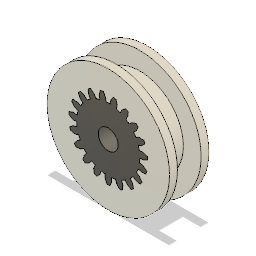
bobin v1 (Autodesk Fusion 360 design; units mm, degrees)
description: Spur Gear; Module: 12.7; Num Teeth: 19; Pressure Angle: 20.0; Backlash: 0.15 mm
Autodesk Fusion 360 part; units mm, degrees
sketch "Sketch1" plane through (0, 0, 0) normal (0, 0, 1) x (1, 0, 0) in component "Spur Gear (19 teeth)"
  circle A0 centre (0, 0) radius 105.3592
  circle A1 centre (0, 0) radius 2.5
extrude "Extrude1" add sketch "Sketch1" along normal blind 10 makes body 1 in component "Spur Gear (19 teeth)"
sketch "Sketch2" plane through (0, 0, 0) normal (0, 0, 1) x (1, 0, 0) in component "Spur Gear (19 teeth)"
  spline S0 degree 5 poles (112.838, -11.0102) (112.8973, -11.0159) (113.0158, -11.0259) (113.1938, -11.0359) (113.4315, -11.04) (113.7289, -11.0326) (114.0267, -11.0162) (114.3246, -10.9942) (114.6226, -10.9694) (114.9207, -10.9425) (115.2187, -10.9134) (115.5167, -10.8815) (115.8147, -10.8457) (116.1127, -10.8055) (116.4106, -10.7609) (116.7084, -10.7123) (117.0062, -10.6603) (117.3038, -10.6054) (117.6013, -10.548) (117.8987, -10.4882) (118.1959, -10.4261) (118.4929, -10.3614) (118.7898, -10.294) (119.0865, -10.2239) (119.3831, -10.1512) (119.6794, -10.0758) (119.9755, -9.9981) (120.2715, -9.918) (120.5672, -9.8357) (120.8627, -9.7512) (121.158, -9.6646) (121.453, -9.5758) (121.7478, -9.4848) (122.0423, -9.3917) (122.3366, -9.2964) (122.6306, -9.199) (122.9244, -9.0996) (123.2178, -8.9982) (123.5111, -8.8949) (123.804, -8.7896) (124.0966, -8.6823) (124.3889, -8.5732) (124.681, -8.4621) (124.9727, -8.3492) (125.2641, -8.2344) (125.5552, -8.1178) (125.846, -7.9993) (126.1365, -7.879) (126.4266, -7.757) (126.7164, -7.6332) (127.0059, -7.5077) (127.295, -7.3804) (127.5837, -7.2514) (127.8722, -7.1207) (128.1602, -6.9883) (128.4479, -6.8542) (128.7353, -6.7185) (129.0222, -6.5811) (129.3088, -6.4421) (129.595, -6.3015) (129.8809, -6.1592) (130.1663, -6.0154) (130.4514, -5.8699) (130.7361, -5.7229) (131.0203, -5.5743) (131.3042, -5.4242) (131.5877, -5.2725) (131.8707, -5.1193) (132.1534, -4.9646) (132.4356, -4.8083) (132.7174, -4.6506) (132.9425, -4.5232) (133.1112, -4.4269) (133.2235, -4.3625) (133.2797, -4.3302) knots 0 0 0 0 0 0 0.01428571 0.02857143 0.04285714 0.05714286 0.07142857 0.08571429 0.1 0.11428571 0.12857143 0.14285714 0.15714286 0.17142857 0.18571429 0.2 0.21428571 0.22857143 0.24285714 0.25714286 0.27142857 0.28571429 0.3 0.31428571 0.32857143 0.34285714 0.35714286 0.37142857 0.38571429 0.4 0.41428571 0.42857143 0.44285714 0.45714286 0.47142857 0.48571429 0.5 0.51428571 0.52857143 0.54285714 0.55714286 0.57142857 0.58571429 0.6 0.61428571 0.62857143 0.64285714 0.65714286 0.67142857 0.68571429 0.7 0.71428571 0.72857143 0.74285714 0.75714286 0.77142857 0.78571429 0.8 0.81428571 0.82857143 0.84285714 0.85714286 0.87142857 0.88571429 0.9 0.91428571 0.92857143 0.94285714 0.95714286 0.97142857 0.98571429 1 1 1 1 1 1
  spline S1 degree 5 poles (112.838, 11.0102) (112.8973, 11.0159) (113.0158, 11.0259) (113.1938, 11.0359) (113.4315, 11.04) (113.7289, 11.0326) (114.0267, 11.0162) (114.3246, 10.9942) (114.6226, 10.9694) (114.9207, 10.9425) (115.2187, 10.9134) (115.5167, 10.8815) (115.8147, 10.8457) (116.1127, 10.8055) (116.4106, 10.7609) (116.7084, 10.7123) (117.0062, 10.6603) (117.3038, 10.6054) (117.6013, 10.548) (117.8987, 10.4882) (118.1959, 10.4261) (118.4929, 10.3614) (118.7898, 10.294) (119.0865, 10.2239) (119.3831, 10.1512) (119.6794, 10.0758) (119.9755, 9.9981) (120.2715, 9.918) (120.5672, 9.8357) (120.8627, 9.7512) (121.158, 9.6646) (121.453, 9.5758) (121.7478, 9.4848) (122.0423, 9.3917) (122.3366, 9.2964) (122.6306, 9.199) (122.9244, 9.0996) (123.2178, 8.9982) (123.5111, 8.8949) (123.804, 8.7896) (124.0966, 8.6823) (124.3889, 8.5732) (124.681, 8.4621) (124.9727, 8.3492) (125.2641, 8.2344) (125.5552, 8.1178) (125.846, 7.9993) (126.1365, 7.879) (126.4266, 7.757) (126.7164, 7.6332) (127.0059, 7.5077) (127.295, 7.3804) (127.5837, 7.2514) (127.8722, 7.1207) (128.1602, 6.9883) (128.4479, 6.8542) (128.7353, 6.7185) (129.0222, 6.5811) (129.3088, 6.4421) (129.595, 6.3015) (129.8809, 6.1592) (130.1663, 6.0154) (130.4514, 5.8699) (130.7361, 5.7229) (131.0203, 5.5743) (131.3042, 5.4242) (131.5877, 5.2725) (131.8707, 5.1193) (132.1534, 4.9646) (132.4356, 4.8083) (132.7174, 4.6506) (132.9425, 4.5232) (133.1112, 4.4269) (133.2235, 4.3625) (133.2797, 4.3302) knots 0 0 0 0 0 0 0.01428571 0.02857143 0.04285714 0.05714286 0.07142857 0.08571429 0.1 0.11428571 0.12857143 0.14285714 0.15714286 0.17142857 0.18571429 0.2 0.21428571 0.22857143 0.24285714 0.25714286 0.27142857 0.28571429 0.3 0.31428571 0.32857143 0.34285714 0.35714286 0.37142857 0.38571429 0.4 0.41428571 0.42857143 0.44285714 0.45714286 0.47142857 0.48571429 0.5 0.51428571 0.52857143 0.54285714 0.55714286 0.57142857 0.58571429 0.6 0.61428571 0.62857143 0.64285714 0.65714286 0.67142857 0.68571429 0.7 0.71428571 0.72857143 0.74285714 0.75714286 0.77142857 0.78571429 0.8 0.81428571 0.82857143 0.84285714 0.85714286 0.87142857 0.88571429 0.9 0.91428571 0.92857143 0.94285714 0.95714286 0.97142857 0.98571429 1 1 1 1 1 1
  arc A0 (133.2797, -4.3302) -> (133.2797, 4.3302) centre (0, 0) ccw
  line L0 (104.8512, -10.2318) -> (112.838, -11.0102)
  line L1 (104.8512, 10.2318) -> (112.838, 11.0102)
  line L2 (104.8512, -10.2318) -> (104.8512, 10.2318)
  point P0 (114.2728, -10.9975)
  point P1 (115.7195, -10.8565)
  point P2 (117.1734, -10.6291)
  point P3 (118.6325, -10.3293)
  point P4 (120.0955, -9.9653)
  point P5 (121.5612, -9.5421)
  point P6 (123.0286, -9.0634)
  point P7 (124.4968, -8.5319)
  point P8 (125.9651, -7.9498)
  point P9 (127.4326, -7.3187)
  point P10 (128.8985, -6.6401)
  point P11 (130.3621, -5.9152)
  point P12 (131.8228, -5.145)
  point P13 (114.2728, 10.9975)
  point P14 (115.7195, 10.8565)
  point P15 (117.1734, 10.6291)
  point P16 (118.6325, 10.3293)
  point P17 (120.0955, 9.9653)
  point P18 (121.5612, 9.5421)
  point P19 (123.0286, 9.0634)
  point P20 (124.4968, 8.5319)
  point P21 (125.9651, 7.9498)
  point P22 (127.4326, 7.3187)
  point P23 (128.8985, 6.6401)
  point P24 (130.3621, 5.9152)
  point P25 (131.8228, 5.145)
extrude "Extrude2" add sketch "Sketch2" along normal blind 10 bodies 1 in component "Spur Gear (19 teeth)"
fillet "Fillet1" radius 0.75 2 edges at (104.8611, -10.2328, 5) (104.8611, 10.2328, 5) on bodies 1 in component "Spur Gear (19 teeth)"
pattern_circular "C-Pattern1" count 19 over 360 about axis through (0, 0, 0) along (0, 0, 1) of "Extrude2", "Fillet1" in component "Spur Gear (19 teeth)"
sketch "Sketch3" plane through (0, 0, 0) normal (0, 0, 1) x (1, 0, 0) in component "Spur Gear (19 teeth)"
  circle A0 centre (0, 0) radius 120.65 construction
sketch "Sketch2 (2)" plane through (0, 0, 0) normal (0, 0, 1) x (1, 0, 0)
  circle A0 centre (0, 66.5) radius 8
  line L0 (0.8502, 58.5453) -> (0.8502, 57.6)
  line L1 (0.8502, 57.6) -> (0.3705, 56.5344)
  line L2 (0.3705, 56.5344) -> (-0.3738, 56.5344)
  line L3 (-0.3738, 56.5344) -> (-0.8, 57.6)
  line L4 (-0.8, 57.6) -> (-0.8, 58.5401)
  line L5 (2.1332, 57.8225) -> (1.8279, 58.7116)
  line L6 (2.8823, 56.953) -> (2.1332, 57.8225)
  line L7 (3.5862, 57.1947) -> (2.8823, 56.953)
  line L8 (3.694, 58.3583) -> (3.5862, 57.1947)
  line L9 (3.3871, 59.2524) -> (3.694, 58.3583)
  line L10 (4.8352, 58.9853) -> (4.2578, 59.7272)
  line L11 (5.826, 58.4062) -> (4.8352, 58.9853)
  line L12 (6.4133, 58.8633) -> (5.826, 58.4062)
  line L13 (6.1375, 59.9989) -> (6.4133, 58.8633)
  line L14 (5.5568, 60.7449) -> (6.1375, 59.9989)
  line L15 (7.0132, 60.9624) -> (6.2262, 61.4766)
  line L16 (8.1384, 60.7364) -> (7.0132, 60.9624)
  line L17 (8.5455, 61.3595) -> (8.1384, 60.7364)
  line L18 (7.9158, 62.344) -> (8.5455, 61.3595)
  line L19 (7.1244, 62.861) -> (7.9158, 62.344)
  line L20 (8.4313, 63.5397) -> (7.5199, 63.7704)
  line L21 (9.5689, 63.6913) -> (8.4313, 63.5397)
  line L22 (9.7516, 64.4127) -> (9.5689, 63.6913)
  line L23 (8.8364, 65.1394) -> (9.7516, 64.4127)
  line L24 (7.92, 65.3715) -> (8.8364, 65.1394)
  line L25 (8.9357, 66.4377) -> (7.9988, 66.3601)
  line L26 (9.9624, 66.9505) -> (8.9357, 66.4377)
  line L27 (9.901, 67.6922) -> (9.9624, 66.9505)
  line L28 (8.7994, 68.0823) -> (9.901, 67.6922)
  line L29 (7.8573, 68.0042) -> (8.7994, 68.0823)
  line L30 (8.4717, 69.3425) -> (7.6108, 68.9648)
  line L31 (9.2764, 70.1608) -> (8.4717, 69.3425)
  line L32 (8.9774, 70.8424) -> (9.2764, 70.1608)
  line L33 (7.8088, 70.8537) -> (8.9774, 70.8424)
  line L34 (6.9432, 70.474) -> (7.8088, 70.8537)
  line L35 (7.0898, 71.9392) -> (6.3981, 71.3025)
  line L36 (7.5851, 72.9745) -> (7.0898, 71.9392)
  line L37 (7.081, 73.5221) -> (7.5851, 72.9745)
  line L38 (5.9721, 73.1534) -> (7.081, 73.5221)
  line L39 (5.2766, 72.5131) -> (5.9721, 73.1534)
  line L40 (4.9395, 73.9466) -> (4.4921, 73.1198)
  line L41 (5.0718, 75.0866) -> (4.9395, 73.9466)
  line L42 (4.4173, 75.4408) -> (5.0718, 75.0866)
  line L43 (3.4882, 74.732) -> (4.4173, 75.4408)
  line L44 (3.0382, 73.9006) -> (3.4882, 74.732)
  line L45 (2.254, 75.1469) -> (2.0992, 74.2197)
  line L46 (2.0089, 76.2682) -> (2.254, 75.1469)
  line L47 (1.2749, 76.3907) -> (2.0089, 76.2682)
  line L48 (0.6262, 75.4186) -> (1.2749, 76.3907)
  line L49 (0.4706, 74.4861) -> (0.6262, 75.4186)
  line L50 (-0.6758, 75.4103) -> (-0.5211, 74.483)
  line L51 (-1.2716, 76.3912) -> (-0.6758, 75.4103)
  line L52 (-2.0057, 76.2687) -> (-1.2716, 76.3912)
  line L53 (-2.3035, 75.1387) -> (-2.0057, 76.2687)
  line L54 (-2.148, 74.2063) -> (-2.3035, 75.1387)
  line L55 (-3.5324, 74.7081) -> (-3.0849, 73.8813)
  line L56 (-4.4144, 75.4424) -> (-3.5324, 74.7081)
  line L57 (-5.0689, 75.0882) -> (-4.4144, 75.4424)
  line L58 (-4.9837, 73.9226) -> (-5.0689, 75.0882)
  line L59 (-4.5338, 73.0913) -> (-4.9837, 73.9226)
  line L60 (-6.0061, 73.1164) -> (-5.3145, 72.4797)
  line L61 (-7.0788, 73.5245) -> (-6.0061, 73.1164)
  line L62 (-7.5828, 72.9769) -> (-7.0788, 73.5245)
  line L63 (-7.1238, 71.9023) -> (-7.5828, 72.9769)
  line L64 (-6.4283, 71.262) -> (-7.1238, 71.9023)
  line L65 (-7.829, 70.8077) -> (-6.9681, 70.4301)
  line L66 (-8.9761, 70.8454) -> (-7.829, 70.8077)
  line L67 (-9.275, 70.1639) -> (-8.9761, 70.8454)
  line L68 (-8.4919, 69.2965) -> (-9.275, 70.1639)
  line L69 (-7.6262, 68.9167) -> (-8.4919, 69.2965)
  line L70 (-8.8035, 68.0322) -> (-7.8666, 67.9546)
  line L71 (-9.9007, 67.6954) -> (-8.8035, 68.0322)
  line L72 (-9.9621, 66.9537) -> (-9.9007, 67.6954)
  line L73 (-8.9398, 66.3876) -> (-9.9621, 66.9537)
  line L74 (-7.9977, 66.3096) -> (-8.9398, 66.3876)
  line L75 (-8.8241, 65.0907) -> (-7.9127, 65.3215)
  line L76 (-9.7524, 64.4159) -> (-8.8241, 65.0907)
  line L77 (-9.5697, 63.6945) -> (-9.7524, 64.4159)
  line L78 (-8.4189, 63.4909) -> (-9.5697, 63.6945)
  line L79 (-7.5026, 63.723) -> (-8.4189, 63.4909)
  line L80 (-7.8883, 62.3019) -> (-7.1013, 62.8161)
  line L81 (-8.5473, 61.3622) -> (-7.8883, 62.3019)
  line L82 (-8.1402, 60.7392) -> (-8.5473, 61.3622)
  line L83 (-6.9857, 60.9204) -> (-8.1402, 60.7392)
  line L84 (-6.1944, 61.4374) -> (-6.9857, 60.9204)
  line L85 (-6.0978, 59.968) -> (-5.5204, 60.7099)
  line L86 (-6.4159, 58.8653) -> (-6.0978, 59.968)
  line L87 (-5.8286, 58.4082) -> (-6.4159, 58.8653)
  line L88 (-4.7955, 58.9544) -> (-5.8286, 58.4082)
  line L89 (-4.2149, 59.7004) -> (-4.7955, 58.9544)
  line L90 (-3.6465, 58.342) -> (-3.3412, 59.2312)
  line L91 (-3.5893, 57.1957) -> (-3.6465, 58.342)
  line L92 (-2.8854, 56.9541) -> (-3.5893, 57.1957)
  line L93 (-2.0856, 57.8062) -> (-2.8854, 56.9541)
  line L94 (-1.7787, 58.7002) -> (-2.0856, 57.8062)
  dimension "d15" = 16
  dimension "d19" = 360
  constraint coincident A0 L0.start
  constraint vertical L0
  constraint perpendicular L0 L2
  constraint coincident A0 L4.end
  constraint perpendicular L2 L4
  measures "d15" diameter of A0
extrude "Extrude1'" add sketch "Sketch2 (2)" along normal blind 10 separate body makes body 2
sketch "Sketch3 (2)" plane through (0, 0, 10) normal (0, 0, 1) x (1, 0, 0)
  arc A0 (0.8502, 58.5453) -> (1.8279, 58.7116) centre (0, 66.5) ccw
  line L0 (1.8279, 58.7116) -> (2.1332, 57.8225)
  line L1 (2.1332, 57.8225) -> (2.8823, 56.953)
  line L2 (2.8823, 56.953) -> (3.5862, 57.1947)
  line L3 (3.5862, 57.1947) -> (3.694, 58.3583)
  line L4 (3.694, 58.3583) -> (3.3871, 59.2524)
  arc A1 (3.3871, 59.2524) -> (4.2578, 59.7272) centre (0, 66.5) ccw
  line L5 (4.2578, 59.7272) -> (4.8352, 58.9853)
  line L6 (4.8352, 58.9853) -> (5.826, 58.4062)
  line L7 (5.826, 58.4062) -> (6.4133, 58.8633)
  line L8 (6.4133, 58.8633) -> (6.1375, 59.9989)
  line L9 (6.1375, 59.9989) -> (5.5568, 60.7449)
  arc A2 (5.5568, 60.7449) -> (6.2262, 61.4766) centre (0, 66.5) ccw
  line L10 (6.2262, 61.4766) -> (7.0132, 60.9624)
  line L11 (7.0132, 60.9624) -> (8.1384, 60.7364)
  line L12 (8.1384, 60.7364) -> (8.5455, 61.3595)
  line L13 (8.5455, 61.3595) -> (7.9158, 62.344)
  line L14 (7.9158, 62.344) -> (7.1244, 62.861)
  arc A3 (7.1244, 62.861) -> (7.5199, 63.7704) centre (0, 66.5) ccw
  line L15 (7.5199, 63.7704) -> (8.4313, 63.5397)
  line L16 (8.4313, 63.5397) -> (9.5689, 63.6913)
  line L17 (9.5689, 63.6913) -> (9.7516, 64.4127)
  line L18 (9.7516, 64.4127) -> (8.8364, 65.1394)
  line L19 (8.8364, 65.1394) -> (7.92, 65.3715)
  arc A4 (7.92, 65.3715) -> (7.9988, 66.3601) centre (0, 66.5) ccw
  line L20 (7.9988, 66.3601) -> (8.9357, 66.4377)
  line L21 (8.9357, 66.4377) -> (9.9624, 66.9505)
  line L22 (9.9624, 66.9505) -> (9.901, 67.6922)
  line L23 (9.901, 67.6922) -> (8.7994, 68.0823)
  line L24 (8.7994, 68.0823) -> (7.8573, 68.0042)
  arc A5 (7.8573, 68.0042) -> (7.6108, 68.9648) centre (0, 66.5) ccw
  line L25 (7.6108, 68.9648) -> (8.4717, 69.3425)
  line L26 (8.4717, 69.3425) -> (9.2764, 70.1608)
  line L27 (9.2764, 70.1608) -> (8.9774, 70.8424)
  line L28 (8.9774, 70.8424) -> (7.8088, 70.8537)
  line L29 (7.8088, 70.8537) -> (6.9432, 70.474)
  arc A6 (6.9432, 70.474) -> (6.3981, 71.3025) centre (0, 66.5) ccw
  line L30 (6.3981, 71.3025) -> (7.0898, 71.9392)
  line L31 (7.0898, 71.9392) -> (7.5851, 72.9745)
  line L32 (7.5851, 72.9745) -> (7.081, 73.5221)
  line L33 (7.081, 73.5221) -> (5.9721, 73.1534)
  line L34 (5.9721, 73.1534) -> (5.2766, 72.5131)
  arc A7 (5.2766, 72.5131) -> (4.4921, 73.1198) centre (0, 66.5) ccw
  line L35 (4.4921, 73.1198) -> (4.9395, 73.9466)
  line L36 (4.9395, 73.9466) -> (5.0718, 75.0866)
  line L37 (5.0718, 75.0866) -> (4.4173, 75.4408)
  line L38 (4.4173, 75.4408) -> (3.4882, 74.732)
  line L39 (3.4882, 74.732) -> (3.0382, 73.9006)
  arc A8 (3.0382, 73.9006) -> (2.0992, 74.2197) centre (0, 66.5) ccw
  line L40 (2.0992, 74.2197) -> (2.254, 75.1469)
  line L41 (2.254, 75.1469) -> (2.0089, 76.2682)
  line L42 (2.0089, 76.2682) -> (1.2749, 76.3907)
  line L43 (1.2749, 76.3907) -> (0.6262, 75.4186)
  line L44 (0.6262, 75.4186) -> (0.4706, 74.4861)
  arc A9 (0.4706, 74.4861) -> (-0.5211, 74.483) centre (0, 66.5) ccw
  line L45 (-0.5211, 74.483) -> (-0.6758, 75.4103)
  line L46 (-0.6758, 75.4103) -> (-1.2716, 76.3912)
  line L47 (-1.2716, 76.3912) -> (-2.0057, 76.2687)
  line L48 (-2.0057, 76.2687) -> (-2.3035, 75.1387)
  line L49 (-2.3035, 75.1387) -> (-2.148, 74.2063)
  arc A10 (-2.148, 74.2063) -> (-3.0849, 73.8813) centre (0, 66.5) ccw
  line L50 (-3.0849, 73.8813) -> (-3.5324, 74.7081)
  line L51 (-3.5324, 74.7081) -> (-4.4144, 75.4424)
  line L52 (-4.4144, 75.4424) -> (-5.0689, 75.0882)
  line L53 (-5.0689, 75.0882) -> (-4.9837, 73.9226)
  line L54 (-4.9837, 73.9226) -> (-4.5338, 73.0913)
  arc A11 (-4.5338, 73.0913) -> (-5.3145, 72.4797) centre (0, 66.5) ccw
  line L55 (-5.3145, 72.4797) -> (-6.0061, 73.1164)
  line L56 (-6.0061, 73.1164) -> (-7.0788, 73.5245)
  line L57 (-7.0788, 73.5245) -> (-7.5828, 72.9769)
  line L58 (-7.5828, 72.9769) -> (-7.1238, 71.9023)
  line L59 (-7.1238, 71.9023) -> (-6.4283, 71.262)
  arc A12 (-6.4283, 71.262) -> (-6.9681, 70.4301) centre (0, 66.5) ccw
  line L60 (-6.9681, 70.4301) -> (-7.829, 70.8077)
  line L61 (-7.829, 70.8077) -> (-8.9761, 70.8454)
  line L62 (-8.9761, 70.8454) -> (-9.275, 70.1639)
  line L63 (-9.275, 70.1639) -> (-8.4919, 69.2965)
  line L64 (-8.4919, 69.2965) -> (-7.6262, 68.9167)
  arc A13 (-7.6262, 68.9167) -> (-7.8666, 67.9546) centre (0, 66.5) ccw
  line L65 (-7.8666, 67.9546) -> (-8.8035, 68.0322)
  line L66 (-8.8035, 68.0322) -> (-9.9007, 67.6954)
  line L67 (-9.9007, 67.6954) -> (-9.9621, 66.9537)
  line L68 (-9.9621, 66.9537) -> (-8.9398, 66.3876)
  line L69 (-8.9398, 66.3876) -> (-7.9977, 66.3096)
  arc A14 (-7.9977, 66.3096) -> (-7.9127, 65.3215) centre (0, 66.5) ccw
  line L70 (-7.9127, 65.3215) -> (-8.8241, 65.0907)
  line L71 (-8.8241, 65.0907) -> (-9.7524, 64.4159)
  line L72 (-9.7524, 64.4159) -> (-9.5697, 63.6945)
  line L73 (-9.5697, 63.6945) -> (-8.4189, 63.4909)
  line L74 (-8.4189, 63.4909) -> (-7.5026, 63.723)
  arc A15 (-7.5026, 63.723) -> (-7.1013, 62.8161) centre (0, 66.5) ccw
  line L75 (-7.1013, 62.8161) -> (-7.8883, 62.3019)
  line L76 (-7.8883, 62.3019) -> (-8.5473, 61.3622)
  line L77 (-8.5473, 61.3622) -> (-8.1402, 60.7392)
  line L78 (-8.1402, 60.7392) -> (-6.9857, 60.9204)
  line L79 (-6.9857, 60.9204) -> (-6.1944, 61.4374)
  arc A16 (-6.1944, 61.4374) -> (-5.5204, 60.7099) centre (0, 66.5) ccw
  line L80 (-5.5204, 60.7099) -> (-6.0978, 59.968)
  line L81 (-6.0978, 59.968) -> (-6.4159, 58.8653)
  line L82 (-6.4159, 58.8653) -> (-5.8286, 58.4082)
  line L83 (-5.8286, 58.4082) -> (-4.7955, 58.9544)
  line L84 (-4.7955, 58.9544) -> (-4.2149, 59.7004)
  arc A17 (-4.2149, 59.7004) -> (-3.3412, 59.2312) centre (0, 66.5) ccw
  line L85 (-3.3412, 59.2312) -> (-3.6465, 58.342)
  line L86 (-3.6465, 58.342) -> (-3.5893, 57.1957)
  line L87 (-3.5893, 57.1957) -> (-2.8854, 56.9541)
  line L88 (-2.8854, 56.9541) -> (-2.0856, 57.8062)
  line L89 (-2.0856, 57.8062) -> (-1.7787, 58.7002)
  arc A18 (-1.7787, 58.7002) -> (-0.8, 58.5401) centre (0, 66.5) ccw
  line L90 (-0.8, 58.5401) -> (-0.8, 57.6)
  line L91 (-0.8, 57.6) -> (-0.3738, 56.5344)
  line L92 (-0.3738, 56.5344) -> (0.3705, 56.5344)
  line L93 (0.3705, 56.5344) -> (0.8502, 57.6)
  line L94 (0.8502, 57.6) -> (0.8502, 58.5453)
  circle A19 centre (0, 66.5) radius 15.5
  circle A20 centre (0, 66.5) radius 11
  dimension "d22" = 31
  dimension "d23" = 22
  constraint concentric A0 A19
  constraint concentric A19 A20
  measures "d22" diameter of A19
  measures "d23" diameter of A20
extrude "Extrude2'" add sketch "Sketch3 (2)" against normal blind 10 separate body contours A20 makes body 3
sketch "Sketch4" plane through (0, 0, 10) normal (0, 0, 1) x (1, 0, 0)
  line L0 (0.8502, 58.5453) -> (0.8502, 57.6)
  line L1 (0.8502, 57.6) -> (0.3705, 56.5344)
  line L2 (0.3705, 56.5344) -> (-0.3738, 56.5344)
  line L3 (-0.3738, 56.5344) -> (-0.8, 57.6)
  line L4 (-0.8, 57.6) -> (-0.8, 58.5401)
  arc A0 (-1.7787, 58.7002) -> (-0.8, 58.5401) centre (0, 66.5) ccw
  line L5 (-1.7787, 58.7002) -> (-2.0856, 57.8062)
  line L6 (-2.0856, 57.8062) -> (-2.8854, 56.9541)
  line L7 (-2.8854, 56.9541) -> (-3.5893, 57.1957)
  line L8 (-3.5893, 57.1957) -> (-3.6465, 58.342)
  line L9 (-3.6465, 58.342) -> (-3.3412, 59.2312)
  arc A1 (-4.2149, 59.7004) -> (-3.3412, 59.2312) centre (0, 66.5) ccw
  line L10 (-4.2149, 59.7004) -> (-4.7955, 58.9544)
  line L11 (-4.7955, 58.9544) -> (-5.8286, 58.4082)
  line L12 (-5.8286, 58.4082) -> (-6.4159, 58.8653)
  line L13 (-6.4159, 58.8653) -> (-6.0978, 59.968)
  line L14 (-6.0978, 59.968) -> (-5.5204, 60.7099)
  arc A2 (-6.1944, 61.4374) -> (-5.5204, 60.7099) centre (0, 66.5) ccw
  line L15 (-6.1944, 61.4374) -> (-6.9857, 60.9204)
  line L16 (-6.9857, 60.9204) -> (-8.1402, 60.7392)
  line L17 (-8.1402, 60.7392) -> (-8.5473, 61.3622)
  line L18 (-8.5473, 61.3622) -> (-7.8883, 62.3019)
  line L19 (-7.8883, 62.3019) -> (-7.1013, 62.8161)
  arc A3 (-7.5026, 63.723) -> (-7.1013, 62.8161) centre (0, 66.5) ccw
  line L20 (-7.5026, 63.723) -> (-8.4189, 63.4909)
  line L21 (-8.4189, 63.4909) -> (-9.5697, 63.6945)
  line L22 (-9.5697, 63.6945) -> (-9.7524, 64.4159)
  line L23 (-9.7524, 64.4159) -> (-8.8241, 65.0907)
  line L24 (-8.8241, 65.0907) -> (-7.9127, 65.3215)
  arc A4 (-7.9977, 66.3096) -> (-7.9127, 65.3215) centre (0, 66.5) ccw
  line L25 (-7.9977, 66.3096) -> (-8.9398, 66.3876)
  line L26 (-8.9398, 66.3876) -> (-9.9621, 66.9537)
  line L27 (-9.9621, 66.9537) -> (-9.9007, 67.6954)
  line L28 (-9.9007, 67.6954) -> (-8.8035, 68.0322)
  line L29 (-8.8035, 68.0322) -> (-7.8666, 67.9546)
  arc A5 (-7.6262, 68.9167) -> (-7.8666, 67.9546) centre (0, 66.5) ccw
  line L30 (-7.6262, 68.9167) -> (-8.4919, 69.2965)
  line L31 (-8.4919, 69.2965) -> (-9.275, 70.1639)
  line L32 (-9.275, 70.1639) -> (-8.9761, 70.8454)
  line L33 (-8.9761, 70.8454) -> (-7.829, 70.8077)
  line L34 (-7.829, 70.8077) -> (-6.9681, 70.4301)
  arc A6 (-6.4283, 71.262) -> (-6.9681, 70.4301) centre (0, 66.5) ccw
  line L35 (-6.4283, 71.262) -> (-7.1238, 71.9023)
  line L36 (-7.1238, 71.9023) -> (-7.5828, 72.9769)
  line L37 (-7.5828, 72.9769) -> (-7.0788, 73.5245)
  line L38 (-7.0788, 73.5245) -> (-6.0061, 73.1164)
  line L39 (-6.0061, 73.1164) -> (-5.3145, 72.4797)
  arc A7 (-4.5338, 73.0913) -> (-5.3145, 72.4797) centre (0, 66.5) ccw
  line L40 (-4.5338, 73.0913) -> (-4.9837, 73.9226)
  line L41 (-4.9837, 73.9226) -> (-5.0689, 75.0882)
  line L42 (-5.0689, 75.0882) -> (-4.4144, 75.4424)
  line L43 (-4.4144, 75.4424) -> (-3.5324, 74.7081)
  line L44 (-3.5324, 74.7081) -> (-3.0849, 73.8813)
  arc A8 (-2.148, 74.2063) -> (-3.0849, 73.8813) centre (0, 66.5) ccw
  line L45 (-2.148, 74.2063) -> (-2.3035, 75.1387)
  line L46 (-2.3035, 75.1387) -> (-2.0057, 76.2687)
  line L47 (-2.0057, 76.2687) -> (-1.2716, 76.3912)
  line L48 (-1.2716, 76.3912) -> (-0.6758, 75.4103)
  line L49 (-0.6758, 75.4103) -> (-0.5211, 74.483)
  arc A9 (0.4706, 74.4861) -> (-0.5211, 74.483) centre (0, 66.5) ccw
  line L50 (0.4706, 74.4861) -> (0.6262, 75.4186)
  line L51 (0.6262, 75.4186) -> (1.2749, 76.3907)
  line L52 (1.2749, 76.3907) -> (2.0089, 76.2682)
  line L53 (2.0089, 76.2682) -> (2.254, 75.1469)
  line L54 (2.254, 75.1469) -> (2.0992, 74.2197)
  arc A10 (3.0382, 73.9006) -> (2.0992, 74.2197) centre (0, 66.5) ccw
  line L55 (3.0382, 73.9006) -> (3.4882, 74.732)
  line L56 (3.4882, 74.732) -> (4.4173, 75.4408)
  line L57 (4.4173, 75.4408) -> (5.0718, 75.0866)
  line L58 (5.0718, 75.0866) -> (4.9395, 73.9466)
  line L59 (4.9395, 73.9466) -> (4.4921, 73.1198)
  arc A11 (5.2766, 72.5131) -> (4.4921, 73.1198) centre (0, 66.5) ccw
  line L60 (5.2766, 72.5131) -> (5.9721, 73.1534)
  line L61 (5.9721, 73.1534) -> (7.081, 73.5221)
  line L62 (7.081, 73.5221) -> (7.5851, 72.9745)
  line L63 (7.5851, 72.9745) -> (7.0898, 71.9392)
  line L64 (7.0898, 71.9392) -> (6.3981, 71.3025)
  arc A12 (6.9432, 70.474) -> (6.3981, 71.3025) centre (0, 66.5) ccw
  line L65 (6.9432, 70.474) -> (7.8088, 70.8537)
  line L66 (7.8088, 70.8537) -> (8.9774, 70.8424)
  line L67 (8.9774, 70.8424) -> (9.2764, 70.1608)
  line L68 (9.2764, 70.1608) -> (8.4717, 69.3425)
  line L69 (8.4717, 69.3425) -> (7.6108, 68.9648)
  arc A13 (7.8573, 68.0042) -> (7.6108, 68.9648) centre (0, 66.5) ccw
  line L70 (7.8573, 68.0042) -> (8.7994, 68.0823)
  line L71 (8.7994, 68.0823) -> (9.901, 67.6922)
  line L72 (9.901, 67.6922) -> (9.9624, 66.9505)
  line L73 (9.9624, 66.9505) -> (8.9357, 66.4377)
  line L74 (8.9357, 66.4377) -> (7.9988, 66.3601)
  arc A14 (7.92, 65.3715) -> (7.9988, 66.3601) centre (0, 66.5) ccw
  line L75 (7.92, 65.3715) -> (8.8364, 65.1394)
  line L76 (8.8364, 65.1394) -> (9.7516, 64.4127)
  line L77 (9.7516, 64.4127) -> (9.5689, 63.6913)
  line L78 (9.5689, 63.6913) -> (8.4313, 63.5397)
  line L79 (8.4313, 63.5397) -> (7.5199, 63.7704)
  arc A15 (7.1244, 62.861) -> (7.5199, 63.7704) centre (0, 66.5) ccw
  line L80 (7.1244, 62.861) -> (7.9158, 62.344)
  line L81 (7.9158, 62.344) -> (8.5455, 61.3595)
  line L82 (8.5455, 61.3595) -> (8.1384, 60.7364)
  line L83 (8.1384, 60.7364) -> (7.0132, 60.9624)
  line L84 (7.0132, 60.9624) -> (6.2262, 61.4766)
  arc A16 (5.5568, 60.7449) -> (6.2262, 61.4766) centre (0, 66.5) ccw
  line L85 (5.5568, 60.7449) -> (6.1375, 59.9989)
  line L86 (6.1375, 59.9989) -> (6.4133, 58.8633)
  line L87 (6.4133, 58.8633) -> (5.826, 58.4062)
  line L88 (5.826, 58.4062) -> (4.8352, 58.9853)
  line L89 (4.8352, 58.9853) -> (4.2578, 59.7272)
  arc A17 (3.3871, 59.2524) -> (4.2578, 59.7272) centre (0, 66.5) ccw
  line L90 (3.3871, 59.2524) -> (3.694, 58.3583)
  line L91 (3.694, 58.3583) -> (3.5862, 57.1947)
  line L92 (3.5862, 57.1947) -> (2.8823, 56.953)
  line L93 (2.8823, 56.953) -> (2.1332, 57.8225)
  line L94 (2.1332, 57.8225) -> (1.8279, 58.7116)
  arc A18 (0.8502, 58.5453) -> (1.8279, 58.7116) centre (0, 66.5) ccw
  circle A19 centre (0, 66.5) radius 11
  circle A20 centre (0, 66.5) radius 15.5
  dimension "d26" = 31
  constraint concentric A0 A20
  measures "d26" diameter of A20
sketch "Sketch5" plane through (0, 0, 0) normal (0, 0, -1) x (-1, 0, 0)
  line L0 (-0.8502, 57.6) -> (-0.8502, 58.5453)
  arc A0 (-1.8279, 58.7116) -> (-0.8502, 58.5453) centre (0, 66.5) ccw
  line L1 (-1.8279, 58.7116) -> (-2.1332, 57.8225)
  line L2 (-2.1332, 57.8225) -> (-2.8823, 56.953)
  line L3 (-2.8823, 56.953) -> (-3.5862, 57.1947)
  line L4 (-3.5862, 57.1947) -> (-3.694, 58.3583)
  line L5 (-3.694, 58.3583) -> (-3.3871, 59.2524)
  arc A1 (-4.2578, 59.7272) -> (-3.3871, 59.2524) centre (0, 66.5) ccw
  line L6 (-4.2578, 59.7272) -> (-4.8352, 58.9853)
  line L7 (-4.8352, 58.9853) -> (-5.826, 58.4062)
  line L8 (-5.826, 58.4062) -> (-6.4133, 58.8633)
  line L9 (-6.4133, 58.8633) -> (-6.1375, 59.9989)
  line L10 (-6.1375, 59.9989) -> (-5.5568, 60.7449)
  arc A2 (-6.2262, 61.4766) -> (-5.5568, 60.7449) centre (0, 66.5) ccw
  line L11 (-6.2262, 61.4766) -> (-7.0132, 60.9624)
  line L12 (-7.0132, 60.9624) -> (-8.1384, 60.7364)
  line L13 (-8.1384, 60.7364) -> (-8.5455, 61.3595)
  line L14 (-8.5455, 61.3595) -> (-7.9158, 62.344)
  line L15 (-7.9158, 62.344) -> (-7.1244, 62.861)
  arc A3 (-7.5199, 63.7704) -> (-7.1244, 62.861) centre (0, 66.5) ccw
  line L16 (-7.5199, 63.7704) -> (-8.4313, 63.5397)
  line L17 (-8.4313, 63.5397) -> (-9.5689, 63.6913)
  line L18 (-9.5689, 63.6913) -> (-9.7516, 64.4127)
  line L19 (-9.7516, 64.4127) -> (-8.8364, 65.1394)
  line L20 (-8.8364, 65.1394) -> (-7.92, 65.3715)
  arc A4 (-7.9988, 66.3601) -> (-7.92, 65.3715) centre (0, 66.5) ccw
  line L21 (-7.9988, 66.3601) -> (-8.9357, 66.4377)
  line L22 (-8.9357, 66.4377) -> (-9.9624, 66.9505)
  line L23 (-9.9624, 66.9505) -> (-9.901, 67.6922)
  line L24 (-9.901, 67.6922) -> (-8.7994, 68.0823)
  line L25 (-8.7994, 68.0823) -> (-7.8573, 68.0042)
  arc A5 (-7.6108, 68.9648) -> (-7.8573, 68.0042) centre (0, 66.5) ccw
  line L26 (-7.6108, 68.9648) -> (-8.4717, 69.3425)
  line L27 (-8.4717, 69.3425) -> (-9.2764, 70.1608)
  line L28 (-9.2764, 70.1608) -> (-8.9774, 70.8424)
  line L29 (-8.9774, 70.8424) -> (-7.8088, 70.8537)
  line L30 (-7.8088, 70.8537) -> (-6.9432, 70.474)
  arc A6 (-6.3981, 71.3025) -> (-6.9432, 70.474) centre (0, 66.5) ccw
  line L31 (-6.3981, 71.3025) -> (-7.0898, 71.9392)
  line L32 (-7.0898, 71.9392) -> (-7.5851, 72.9745)
  line L33 (-7.5851, 72.9745) -> (-7.081, 73.5221)
  line L34 (-7.081, 73.5221) -> (-5.9721, 73.1534)
  line L35 (-5.9721, 73.1534) -> (-5.2766, 72.5131)
  arc A7 (-4.4921, 73.1198) -> (-5.2766, 72.5131) centre (0, 66.5) ccw
  line L36 (-4.4921, 73.1198) -> (-4.9395, 73.9466)
  line L37 (-4.9395, 73.9466) -> (-5.0718, 75.0866)
  line L38 (-5.0718, 75.0866) -> (-4.4173, 75.4408)
  line L39 (-4.4173, 75.4408) -> (-3.4882, 74.732)
  line L40 (-3.4882, 74.732) -> (-3.0382, 73.9006)
  arc A8 (-2.0992, 74.2197) -> (-3.0382, 73.9006) centre (0, 66.5) ccw
  line L41 (-2.0992, 74.2197) -> (-2.254, 75.1469)
  line L42 (-2.254, 75.1469) -> (-2.0089, 76.2682)
  line L43 (-2.0089, 76.2682) -> (-1.2749, 76.3907)
  line L44 (-1.2749, 76.3907) -> (-0.6262, 75.4186)
  line L45 (-0.6262, 75.4186) -> (-0.4706, 74.4861)
  arc A9 (0.5211, 74.483) -> (-0.4706, 74.4861) centre (0, 66.5) ccw
  line L46 (0.5211, 74.483) -> (0.6758, 75.4103)
  line L47 (0.6758, 75.4103) -> (1.2716, 76.3912)
  line L48 (1.2716, 76.3912) -> (2.0057, 76.2687)
  line L49 (2.0057, 76.2687) -> (2.3035, 75.1387)
  line L50 (2.3035, 75.1387) -> (2.148, 74.2063)
  arc A10 (3.0849, 73.8813) -> (2.148, 74.2063) centre (0, 66.5) ccw
  line L51 (3.0849, 73.8813) -> (3.5324, 74.7081)
  line L52 (3.5324, 74.7081) -> (4.4144, 75.4424)
  line L53 (4.4144, 75.4424) -> (5.0689, 75.0882)
  line L54 (5.0689, 75.0882) -> (4.9837, 73.9226)
  line L55 (4.9837, 73.9226) -> (4.5338, 73.0913)
  arc A11 (5.3145, 72.4797) -> (4.5338, 73.0913) centre (0, 66.5) ccw
  line L56 (5.3145, 72.4797) -> (6.0061, 73.1164)
  line L57 (6.0061, 73.1164) -> (7.0788, 73.5245)
  line L58 (7.0788, 73.5245) -> (7.5828, 72.9769)
  line L59 (7.5828, 72.9769) -> (7.1238, 71.9023)
  line L60 (7.1238, 71.9023) -> (6.4283, 71.262)
  arc A12 (6.9681, 70.4301) -> (6.4283, 71.262) centre (0, 66.5) ccw
  line L61 (6.9681, 70.4301) -> (7.829, 70.8077)
  line L62 (7.829, 70.8077) -> (8.9761, 70.8454)
  line L63 (8.9761, 70.8454) -> (9.275, 70.1639)
  line L64 (9.275, 70.1639) -> (8.4919, 69.2965)
  line L65 (8.4919, 69.2965) -> (7.6262, 68.9167)
  arc A13 (7.8666, 67.9546) -> (7.6262, 68.9167) centre (0, 66.5) ccw
  line L66 (7.8666, 67.9546) -> (8.8035, 68.0322)
  line L67 (8.8035, 68.0322) -> (9.9007, 67.6954)
  line L68 (9.9007, 67.6954) -> (9.9621, 66.9537)
  line L69 (9.9621, 66.9537) -> (8.9398, 66.3876)
  line L70 (8.9398, 66.3876) -> (7.9977, 66.3096)
  arc A14 (7.9127, 65.3215) -> (7.9977, 66.3096) centre (0, 66.5) ccw
  line L71 (7.9127, 65.3215) -> (8.8241, 65.0907)
  line L72 (8.8241, 65.0907) -> (9.7524, 64.4159)
  line L73 (9.7524, 64.4159) -> (9.5697, 63.6945)
  line L74 (9.5697, 63.6945) -> (8.4189, 63.4909)
  line L75 (8.4189, 63.4909) -> (7.5026, 63.723)
  arc A15 (7.1013, 62.8161) -> (7.5026, 63.723) centre (0, 66.5) ccw
  line L76 (7.1013, 62.8161) -> (7.8883, 62.3019)
  line L77 (7.8883, 62.3019) -> (8.5473, 61.3622)
  line L78 (8.5473, 61.3622) -> (8.1402, 60.7392)
  line L79 (8.1402, 60.7392) -> (6.9857, 60.9204)
  line L80 (6.9857, 60.9204) -> (6.1944, 61.4374)
  arc A16 (5.5204, 60.7099) -> (6.1944, 61.4374) centre (0, 66.5) ccw
  line L81 (5.5204, 60.7099) -> (6.0978, 59.968)
  line L82 (6.0978, 59.968) -> (6.4159, 58.8653)
  line L83 (6.4159, 58.8653) -> (5.8286, 58.4082)
  line L84 (5.8286, 58.4082) -> (4.7955, 58.9544)
  line L85 (4.7955, 58.9544) -> (4.2149, 59.7004)
  arc A17 (3.3412, 59.2312) -> (4.2149, 59.7004) centre (0, 66.5) ccw
  line L86 (3.3412, 59.2312) -> (3.6465, 58.342)
  line L87 (3.6465, 58.342) -> (3.5893, 57.1957)
  line L88 (3.5893, 57.1957) -> (2.8854, 56.9541)
  line L89 (2.8854, 56.9541) -> (2.0856, 57.8062)
  line L90 (2.0856, 57.8062) -> (1.7787, 58.7002)
  arc A18 (0.8, 58.5401) -> (1.7787, 58.7002) centre (0, 66.5) ccw
  line L91 (0.8, 58.5401) -> (0.8, 57.6)
  line L92 (0.8, 57.6) -> (0.3738, 56.5344)
  line L93 (0.3738, 56.5344) -> (-0.3705, 56.5344)
  line L94 (-0.3705, 56.5344) -> (-0.8502, 57.6)
  circle A19 centre (0, 66.5) radius 11
  circle A20 centre (0, 66.5) radius 15.5
  dimension "d27" = 31
  constraint concentric A0 A20
  measures "d27" diameter of A20
extrude "Extrude3" add sketch "Sketch4" against normal blind 2 contours A20 bodies 3
extrude "Extrude4" add sketch "Sketch5" against normal blind 2 contours A20 bodies 3
sketch "Sketch6" plane through (0, 0, 0) normal (0, 0, -1) x (-1, 0, 0)
  circle A0 centre (0, 66.5) radius 15.5
  line L0 (-0.8502, 57.6) -> (-0.8502, 58.5453)
  arc A1 (-1.8279, 58.7116) -> (-0.8502, 58.5453) centre (0, 66.5) ccw
  line L1 (-1.8279, 58.7116) -> (-2.1332, 57.8225)
  line L2 (-2.1332, 57.8225) -> (-2.8823, 56.953)
  line L3 (-2.8823, 56.953) -> (-3.5862, 57.1947)
  line L4 (-3.5862, 57.1947) -> (-3.694, 58.3583)
  line L5 (-3.694, 58.3583) -> (-3.3871, 59.2524)
  arc A2 (-4.2578, 59.7272) -> (-3.3871, 59.2524) centre (0, 66.5) ccw
  line L6 (-4.2578, 59.7272) -> (-4.8352, 58.9853)
  line L7 (-4.8352, 58.9853) -> (-5.826, 58.4062)
  line L8 (-5.826, 58.4062) -> (-6.4133, 58.8633)
  line L9 (-6.4133, 58.8633) -> (-6.1375, 59.9989)
  line L10 (-6.1375, 59.9989) -> (-5.5568, 60.7449)
  arc A3 (-6.2262, 61.4766) -> (-5.5568, 60.7449) centre (0, 66.5) ccw
  line L11 (-6.2262, 61.4766) -> (-7.0132, 60.9624)
  line L12 (-7.0132, 60.9624) -> (-8.1384, 60.7364)
  line L13 (-8.1384, 60.7364) -> (-8.5455, 61.3595)
  line L14 (-8.5455, 61.3595) -> (-7.9158, 62.344)
  line L15 (-7.9158, 62.344) -> (-7.1244, 62.861)
  arc A4 (-7.5199, 63.7704) -> (-7.1244, 62.861) centre (0, 66.5) ccw
  line L16 (-7.5199, 63.7704) -> (-8.4313, 63.5397)
  line L17 (-8.4313, 63.5397) -> (-9.5689, 63.6913)
  line L18 (-9.5689, 63.6913) -> (-9.7516, 64.4127)
  line L19 (-9.7516, 64.4127) -> (-8.8364, 65.1394)
  line L20 (-8.8364, 65.1394) -> (-7.92, 65.3715)
  arc A5 (-7.9988, 66.3601) -> (-7.92, 65.3715) centre (0, 66.5) ccw
  line L21 (-7.9988, 66.3601) -> (-8.9357, 66.4377)
  line L22 (-8.9357, 66.4377) -> (-9.9624, 66.9505)
  line L23 (-9.9624, 66.9505) -> (-9.901, 67.6922)
  line L24 (-9.901, 67.6922) -> (-8.7994, 68.0823)
  line L25 (-8.7994, 68.0823) -> (-7.8573, 68.0042)
  arc A6 (-7.6108, 68.9648) -> (-7.8573, 68.0042) centre (0, 66.5) ccw
  line L26 (-7.6108, 68.9648) -> (-8.4717, 69.3425)
  line L27 (-8.4717, 69.3425) -> (-9.2764, 70.1608)
  line L28 (-9.2764, 70.1608) -> (-8.9774, 70.8424)
  line L29 (-8.9774, 70.8424) -> (-7.8088, 70.8537)
  line L30 (-7.8088, 70.8537) -> (-6.9432, 70.474)
  arc A7 (-6.3981, 71.3025) -> (-6.9432, 70.474) centre (0, 66.5) ccw
  line L31 (-6.3981, 71.3025) -> (-7.0898, 71.9392)
  line L32 (-7.0898, 71.9392) -> (-7.5851, 72.9745)
  line L33 (-7.5851, 72.9745) -> (-7.081, 73.5221)
  line L34 (-7.081, 73.5221) -> (-5.9721, 73.1534)
  line L35 (-5.9721, 73.1534) -> (-5.2766, 72.5131)
  arc A8 (-4.4921, 73.1198) -> (-5.2766, 72.5131) centre (0, 66.5) ccw
  line L36 (-4.4921, 73.1198) -> (-4.9395, 73.9466)
  line L37 (-4.9395, 73.9466) -> (-5.0718, 75.0866)
  line L38 (-5.0718, 75.0866) -> (-4.4173, 75.4408)
  line L39 (-4.4173, 75.4408) -> (-3.4882, 74.732)
  line L40 (-3.4882, 74.732) -> (-3.0382, 73.9006)
  arc A9 (-2.0992, 74.2197) -> (-3.0382, 73.9006) centre (0, 66.5) ccw
  line L41 (-2.0992, 74.2197) -> (-2.254, 75.1469)
  line L42 (-2.254, 75.1469) -> (-2.0089, 76.2682)
  line L43 (-2.0089, 76.2682) -> (-1.2749, 76.3907)
  line L44 (-1.2749, 76.3907) -> (-0.6262, 75.4186)
  line L45 (-0.6262, 75.4186) -> (-0.4706, 74.4861)
  arc A10 (0.5211, 74.483) -> (-0.4706, 74.4861) centre (0, 66.5) ccw
  line L46 (0.5211, 74.483) -> (0.6758, 75.4103)
  line L47 (0.6758, 75.4103) -> (1.2716, 76.3912)
  line L48 (1.2716, 76.3912) -> (2.0057, 76.2687)
  line L49 (2.0057, 76.2687) -> (2.3035, 75.1387)
  line L50 (2.3035, 75.1387) -> (2.148, 74.2063)
  arc A11 (3.0849, 73.8813) -> (2.148, 74.2063) centre (0, 66.5) ccw
  line L51 (3.0849, 73.8813) -> (3.5324, 74.7081)
  line L52 (3.5324, 74.7081) -> (4.4144, 75.4424)
  line L53 (4.4144, 75.4424) -> (5.0689, 75.0882)
  line L54 (5.0689, 75.0882) -> (4.9837, 73.9226)
  line L55 (4.9837, 73.9226) -> (4.5338, 73.0913)
  arc A12 (5.3145, 72.4797) -> (4.5338, 73.0913) centre (0, 66.5) ccw
  line L56 (5.3145, 72.4797) -> (6.0061, 73.1164)
  line L57 (6.0061, 73.1164) -> (7.0788, 73.5245)
  line L58 (7.0788, 73.5245) -> (7.5828, 72.9769)
  line L59 (7.5828, 72.9769) -> (7.1238, 71.9023)
  line L60 (7.1238, 71.9023) -> (6.4283, 71.262)
  arc A13 (6.9681, 70.4301) -> (6.4283, 71.262) centre (0, 66.5) ccw
  line L61 (6.9681, 70.4301) -> (7.829, 70.8077)
  line L62 (7.829, 70.8077) -> (8.9761, 70.8454)
  line L63 (8.9761, 70.8454) -> (9.275, 70.1639)
  line L64 (9.275, 70.1639) -> (8.4919, 69.2965)
  line L65 (8.4919, 69.2965) -> (7.6262, 68.9167)
  arc A14 (7.8666, 67.9546) -> (7.6262, 68.9167) centre (0, 66.5) ccw
  line L66 (7.8666, 67.9546) -> (8.8035, 68.0322)
  line L67 (8.8035, 68.0322) -> (9.9007, 67.6954)
  line L68 (9.9007, 67.6954) -> (9.9621, 66.9537)
  line L69 (9.9621, 66.9537) -> (8.9398, 66.3876)
  line L70 (8.9398, 66.3876) -> (7.9977, 66.3096)
  arc A15 (7.9127, 65.3215) -> (7.9977, 66.3096) centre (0, 66.5) ccw
  line L71 (7.9127, 65.3215) -> (8.8241, 65.0907)
  line L72 (8.8241, 65.0907) -> (9.7524, 64.4159)
  line L73 (9.7524, 64.4159) -> (9.5697, 63.6945)
  line L74 (9.5697, 63.6945) -> (8.4189, 63.4909)
  line L75 (8.4189, 63.4909) -> (7.5026, 63.723)
  arc A16 (7.1013, 62.8161) -> (7.5026, 63.723) centre (0, 66.5) ccw
  line L76 (7.1013, 62.8161) -> (7.8883, 62.3019)
  line L77 (7.8883, 62.3019) -> (8.5473, 61.3622)
  line L78 (8.5473, 61.3622) -> (8.1402, 60.7392)
  line L79 (8.1402, 60.7392) -> (6.9857, 60.9204)
  line L80 (6.9857, 60.9204) -> (6.1944, 61.4374)
  arc A17 (5.5204, 60.7099) -> (6.1944, 61.4374) centre (0, 66.5) ccw
  line L81 (5.5204, 60.7099) -> (6.0978, 59.968)
  line L82 (6.0978, 59.968) -> (6.4159, 58.8653)
  line L83 (6.4159, 58.8653) -> (5.8286, 58.4082)
  line L84 (5.8286, 58.4082) -> (4.7955, 58.9544)
  line L85 (4.7955, 58.9544) -> (4.2149, 59.7004)
  arc A18 (3.3412, 59.2312) -> (4.2149, 59.7004) centre (0, 66.5) ccw
  line L86 (3.3412, 59.2312) -> (3.6465, 58.342)
  line L87 (3.6465, 58.342) -> (3.5893, 57.1957)
  line L88 (3.5893, 57.1957) -> (2.8854, 56.9541)
  line L89 (2.8854, 56.9541) -> (2.0856, 57.8062)
  line L90 (2.0856, 57.8062) -> (1.7787, 58.7002)
  arc A19 (0.8, 58.5401) -> (1.7787, 58.7002) centre (0, 66.5) ccw
  line L91 (0.8, 58.5401) -> (0.8, 57.6)
  line L92 (0.8, 57.6) -> (0.3738, 56.5344)
  line L93 (0.3738, 56.5344) -> (-0.3705, 56.5344)
  line L94 (-0.3705, 56.5344) -> (-0.8502, 57.6)
sketch "Sketch7" plane through (0, 0, 10) normal (0, 0, 1) x (1, 0, 0)
  arc A0 (0.8502, 58.5453) -> (1.8279, 58.7116) centre (0, 66.5) ccw
  line L0 (1.8279, 58.7116) -> (2.1332, 57.8225)
  line L1 (2.1332, 57.8225) -> (2.8823, 56.953)
  line L2 (2.8823, 56.953) -> (3.5862, 57.1947)
  line L3 (3.5862, 57.1947) -> (3.694, 58.3583)
  line L4 (3.694, 58.3583) -> (3.3871, 59.2524)
  arc A1 (3.3871, 59.2524) -> (4.2578, 59.7272) centre (0, 66.5) ccw
  line L5 (4.2578, 59.7272) -> (4.8352, 58.9853)
  line L6 (4.8352, 58.9853) -> (5.826, 58.4062)
  line L7 (5.826, 58.4062) -> (6.4133, 58.8633)
  line L8 (6.4133, 58.8633) -> (6.1375, 59.9989)
  line L9 (6.1375, 59.9989) -> (5.5568, 60.7449)
  arc A2 (5.5568, 60.7449) -> (6.2262, 61.4766) centre (0, 66.5) ccw
  line L10 (6.2262, 61.4766) -> (7.0132, 60.9624)
  line L11 (7.0132, 60.9624) -> (8.1384, 60.7364)
  line L12 (8.1384, 60.7364) -> (8.5455, 61.3595)
  line L13 (8.5455, 61.3595) -> (7.9158, 62.344)
  line L14 (7.9158, 62.344) -> (7.1244, 62.861)
  arc A3 (7.1244, 62.861) -> (7.5199, 63.7704) centre (0, 66.5) ccw
  line L15 (7.5199, 63.7704) -> (8.4313, 63.5397)
  line L16 (8.4313, 63.5397) -> (9.5689, 63.6913)
  line L17 (9.5689, 63.6913) -> (9.7516, 64.4127)
  line L18 (9.7516, 64.4127) -> (8.8364, 65.1394)
  line L19 (8.8364, 65.1394) -> (7.92, 65.3715)
  arc A4 (7.92, 65.3715) -> (7.9988, 66.3601) centre (0, 66.5) ccw
  line L20 (7.9988, 66.3601) -> (8.9357, 66.4377)
  line L21 (8.9357, 66.4377) -> (9.9624, 66.9505)
  line L22 (9.9624, 66.9505) -> (9.901, 67.6922)
  line L23 (9.901, 67.6922) -> (8.7994, 68.0823)
  line L24 (8.7994, 68.0823) -> (7.8573, 68.0042)
  arc A5 (7.8573, 68.0042) -> (7.6108, 68.9648) centre (0, 66.5) ccw
  line L25 (7.6108, 68.9648) -> (8.4717, 69.3425)
  line L26 (8.4717, 69.3425) -> (9.2764, 70.1608)
  line L27 (9.2764, 70.1608) -> (8.9774, 70.8424)
  line L28 (8.9774, 70.8424) -> (7.8088, 70.8537)
  line L29 (7.8088, 70.8537) -> (6.9432, 70.474)
  arc A6 (6.9432, 70.474) -> (6.3981, 71.3025) centre (0, 66.5) ccw
  line L30 (6.3981, 71.3025) -> (7.0898, 71.9392)
  line L31 (7.0898, 71.9392) -> (7.5851, 72.9745)
  line L32 (7.5851, 72.9745) -> (7.081, 73.5221)
  line L33 (7.081, 73.5221) -> (5.9721, 73.1534)
  line L34 (5.9721, 73.1534) -> (5.2766, 72.5131)
  arc A7 (5.2766, 72.5131) -> (4.4921, 73.1198) centre (0, 66.5) ccw
  line L35 (4.4921, 73.1198) -> (4.9395, 73.9466)
  line L36 (4.9395, 73.9466) -> (5.0718, 75.0866)
  line L37 (5.0718, 75.0866) -> (4.4173, 75.4408)
  line L38 (4.4173, 75.4408) -> (3.4882, 74.732)
  line L39 (3.4882, 74.732) -> (3.0382, 73.9006)
  arc A8 (3.0382, 73.9006) -> (2.0992, 74.2197) centre (0, 66.5) ccw
  line L40 (2.0992, 74.2197) -> (2.254, 75.1469)
  line L41 (2.254, 75.1469) -> (2.0089, 76.2682)
  line L42 (2.0089, 76.2682) -> (1.2749, 76.3907)
  line L43 (1.2749, 76.3907) -> (0.6262, 75.4186)
  line L44 (0.6262, 75.4186) -> (0.4706, 74.4861)
  arc A9 (0.4706, 74.4861) -> (-0.5211, 74.483) centre (0, 66.5) ccw
  line L45 (-0.5211, 74.483) -> (-0.6758, 75.4103)
  line L46 (-0.6758, 75.4103) -> (-1.2716, 76.3912)
  line L47 (-1.2716, 76.3912) -> (-2.0057, 76.2687)
  line L48 (-2.0057, 76.2687) -> (-2.3035, 75.1387)
  line L49 (-2.3035, 75.1387) -> (-2.148, 74.2063)
  arc A10 (-2.148, 74.2063) -> (-3.0849, 73.8813) centre (0, 66.5) ccw
  line L50 (-3.0849, 73.8813) -> (-3.5324, 74.7081)
  line L51 (-3.5324, 74.7081) -> (-4.4144, 75.4424)
  line L52 (-4.4144, 75.4424) -> (-5.0689, 75.0882)
  line L53 (-5.0689, 75.0882) -> (-4.9837, 73.9226)
  line L54 (-4.9837, 73.9226) -> (-4.5338, 73.0913)
  arc A11 (-4.5338, 73.0913) -> (-5.3145, 72.4797) centre (0, 66.5) ccw
  line L55 (-5.3145, 72.4797) -> (-6.0061, 73.1164)
  line L56 (-6.0061, 73.1164) -> (-7.0788, 73.5245)
  line L57 (-7.0788, 73.5245) -> (-7.5828, 72.9769)
  line L58 (-7.5828, 72.9769) -> (-7.1238, 71.9023)
  line L59 (-7.1238, 71.9023) -> (-6.4283, 71.262)
  arc A12 (-6.4283, 71.262) -> (-6.9681, 70.4301) centre (0, 66.5) ccw
  line L60 (-6.9681, 70.4301) -> (-7.829, 70.8077)
  line L61 (-7.829, 70.8077) -> (-8.9761, 70.8454)
  line L62 (-8.9761, 70.8454) -> (-9.275, 70.1639)
  line L63 (-9.275, 70.1639) -> (-8.4919, 69.2965)
  line L64 (-8.4919, 69.2965) -> (-7.6262, 68.9167)
  arc A13 (-7.6262, 68.9167) -> (-7.8666, 67.9546) centre (0, 66.5) ccw
  line L65 (-7.8666, 67.9546) -> (-8.8035, 68.0322)
  line L66 (-8.8035, 68.0322) -> (-9.9007, 67.6954)
  line L67 (-9.9007, 67.6954) -> (-9.9621, 66.9537)
  line L68 (-9.9621, 66.9537) -> (-8.9398, 66.3876)
  line L69 (-8.9398, 66.3876) -> (-7.9977, 66.3096)
  arc A14 (-7.9977, 66.3096) -> (-7.9127, 65.3215) centre (0, 66.5) ccw
  line L70 (-7.9127, 65.3215) -> (-8.8241, 65.0907)
  line L71 (-8.8241, 65.0907) -> (-9.7524, 64.4159)
  line L72 (-9.7524, 64.4159) -> (-9.5697, 63.6945)
  line L73 (-9.5697, 63.6945) -> (-8.4189, 63.4909)
  line L74 (-8.4189, 63.4909) -> (-7.5026, 63.723)
  arc A15 (-7.5026, 63.723) -> (-7.1013, 62.8161) centre (0, 66.5) ccw
  line L75 (-7.1013, 62.8161) -> (-7.8883, 62.3019)
  line L76 (-7.8883, 62.3019) -> (-8.5473, 61.3622)
  line L77 (-8.5473, 61.3622) -> (-8.1402, 60.7392)
  line L78 (-8.1402, 60.7392) -> (-6.9857, 60.9204)
  line L79 (-6.9857, 60.9204) -> (-6.1944, 61.4374)
  arc A16 (-6.1944, 61.4374) -> (-5.5204, 60.7099) centre (0, 66.5) ccw
  line L80 (-5.5204, 60.7099) -> (-6.0978, 59.968)
  line L81 (-6.0978, 59.968) -> (-6.4159, 58.8653)
  line L82 (-6.4159, 58.8653) -> (-5.8286, 58.4082)
  line L83 (-5.8286, 58.4082) -> (-4.7955, 58.9544)
  line L84 (-4.7955, 58.9544) -> (-4.2149, 59.7004)
  arc A17 (-4.2149, 59.7004) -> (-3.3412, 59.2312) centre (0, 66.5) ccw
  line L85 (-3.3412, 59.2312) -> (-3.6465, 58.342)
  line L86 (-3.6465, 58.342) -> (-3.5893, 57.1957)
  line L87 (-3.5893, 57.1957) -> (-2.8854, 56.9541)
  line L88 (-2.8854, 56.9541) -> (-2.0856, 57.8062)
  line L89 (-2.0856, 57.8062) -> (-1.7787, 58.7002)
  arc A18 (-1.7787, 58.7002) -> (-0.8, 58.5401) centre (0, 66.5) ccw
  line L90 (-0.8, 58.5401) -> (-0.8, 57.6)
  line L91 (-0.8, 57.6) -> (-0.3738, 56.5344)
  line L92 (-0.3738, 56.5344) -> (0.3705, 56.5344)
  line L93 (0.3705, 56.5344) -> (0.8502, 57.6)
  line L94 (0.8502, 57.6) -> (0.8502, 58.5453)
  circle A19 centre (0, 66.5) radius 2.5
  dimension "d32" = 5
  constraint concentric A0 A19
  measures "d32" diameter of A19
extrude "Extrude5" cut sketch "Sketch7" against normal through all contours A19 bodies 2
component "Spur Gear (19 teeth)" placed x (1, 0, 0) y (0, 1, 0) z (0, 0, 1) at (0, 0, 0)
